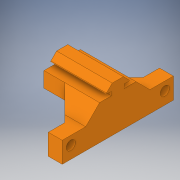
# Autodesk Inventor part: 20X20 lift conecter
Saved by Autodesk Inventor 2019 (Build 230136000, 136)
## iProperties
Created: 2018-10-23
Part Number: 20X20 lift conecter
Material: PC/ABS Plastic
Document SubType Name: Modeling
Designer: User
Density: 0.357273 g/cm^3
Appearance: Orange
Mass: 2.99758 g
Surface Area: 36.2331 cm^2
Volume: 8.39019 cm^3
Author: User
Autodesk Inventor part; units mm, degrees
ref_plane "YZ Plane" through (0, 0, 0) normal (1, 0, 0) x (0, 1, 0)
ref_plane "XZ Plane" through (0, 0, 0) normal (0, 1, 0) x (-1, 0, 0)
ref_plane "XY Plane" through (0, 0, 0) normal (0, 0, 1) x (1, 0, 0)
sketch "Sketch1" plane through (0, 0, 0) normal (0, 1, 0) x (-1, 0, 0)
  line L0 (2.54, 0) -> (5.715, 0)
  line L1 (5.715, 0) -> (5.715, -16.637)
  line L2 (5.715, -16.637) -> (2.54, -16.637)
  line L3 (2.54, -5.3975) -> (7.493, -5.3975)
  line L4 (7.493, -5.3975) -> (7.493, -11.2395)
  line L5 (7.493, -11.2395) -> (2.54, -11.2395)
  line L6 (10.5664, -5.7785) -> (10.5664, -10.8585)
  line L7 (7.493, -13.9319) -> (7.493, -2.7051)
  line L8 (7.493, -13.9319) -> (10.5664, -10.8585)
  line L9 (7.493, -2.7051) -> (10.5664, -5.7785)
  line L10 (2.54, -16.637) -> (2.54, 0)
  point P0 (0, 0)
  dimension "d1" = 16.637
  dimension "d2" = 1.778
  dimension "d9" = 3.0734
  dimension "d12" = 0
  dimension "d16" = 11.2268
  dimension "d20" = 135
  dimension "d21" = 135
  dimension "d26" = 2.6924
  dimension "d38" = 5.08
  dimension "d77" = 5.842
  dimension "d78" = 5.3975
  constraints: 22 end point, 3 parallel, 2 horizontal, 2 perpendicular, 2 point on line
  measures "d1" distance of L0.end L1.end
  measures "d2" distance between parallel lines of L4 L1
  measures "d9" distance between parallel lines of L6 L7
  measures "d12" distance between parallel lines of L4 L7
  measures "d16" distance of L7.start L7.end
  measures "d20" angle of L8 L6
  measures "d21" angle of L9 L6
  measures "d26" distance from line of L3 L7.end
  measures "d38" distance of L6.start L6.end
  measures "d77" distance between parallel lines of L5 L3
  measures "d78" distance between parallel lines of L2 L5
extrude "Extrusion2" add sketch "Sketch1" along normal blind 25.4
fillet "Fillet1" radius 0.254 2 edges at (-7.493, 12.7, -13.9319) (-7.493, 12.7, -2.7051)
thicken "Thicken1" operation add thickness 3.81 both sides no extend neighbours yes toward (1, 0, 0) faces at (-2.54, 8.4667, -5.5457)
sketch "Sketch2" plane through (0, 25.4, 0) normal (0, 1, 0) x (1, 0, 0)
  line L0 (-5.715, 5.3975) -> (-5.715, 0) projected
  line L1 (-5.715, 16.637) -> (-5.715, 11.2395) projected
  line L2 (-5.715, 0) -> (10.16, 0)
  line L3 (10.16, 0) -> (10.16, 16.637)
  line L4 (10.16, 16.637) -> (-5.715, 16.637)
  line L5 (-5.715, 16.637) -> (-5.715, 0)
  point P0 (0, 0)
  dimension "d46" = 15.875
  constraints: 8 end point, 2 parallel, 1 horizontal, 1 perpendicular
  measures "d46" distance of L4.end L3.end
extrude "Extrusion3" add sketch "Sketch2" against normal blind 6.35
sketch "Sketch3" plane through (0, 25.4, 0) normal (0, 1, 0) x (1, 0, 0)
  line L0 (0.635, -17.0815) -> (10.16, -17.0815)
  line L1 (10.16, -17.0815) -> (10.16, 33.7185)
  line L2 (10.16, 33.7185) -> (0.635, 33.7185)
  line L3 (0.635, 33.7185) -> (0.635, -17.0815)
  line L4 (10.16, 0) -> (10.16, 16.637) projected
  line L5 (-5.715, 11.2395) -> (-7.493, 11.2395) projected
  line L6 (-7.493, 11.2395) -> (-7.493, 13.3187) projected
  arc A0 (-7.493, 13.3187) -> (-7.9266, 13.4983) centre (-7.747, 13.3187) ccw projected
  line L7 (-7.9266, 13.4983) -> (-10.5664, 10.8585) projected
  line L8 (-10.5664, 10.8585) -> (-10.5664, 5.7785) projected
  line L9 (-10.5664, 5.7785) -> (-7.9266, 3.1387) projected
  arc A1 (-7.9266, 3.1387) -> (-7.493, 3.3183) centre (-7.747, 3.3183) ccw projected
  line L10 (-7.493, 3.3183) -> (-7.493, 5.3975) projected
  line L11 (-7.493, 5.3975) -> (-5.715, 5.3975) projected
  line L12 (-5.715, 5.3975) -> (-5.715, 0) projected
  line L13 (-5.715, 0) -> (10.16, 0) projected
  line L14 (10.16, 0) -> (10.16, 16.637) projected
  line L15 (10.16, 16.637) -> (-5.715, 16.637) projected
  line L16 (-5.715, 16.637) -> (-5.715, 11.2395) projected
  point P0 (0, 0)
  dimension "d49" = 50.8
  dimension "d50" = 16.637
  dimension "d51" = 17.0815
  dimension "d52" = 9.525
  constraints: 8 end point, 2 parallel, 1 collinear, 1 horizontal, 1 perpendicular
  measures "d49" distance of L0.end L1.end
  measures "d50" distance between parallel lines of L15 L13
  measures "d51" distance between parallel lines of L13 L0
  measures "d52" distance of L1.end L2.end
extrude "Extrusion4" add sketch "Sketch3" against normal blind 6.35 contours L3 L13 L1 L0 | L3 L15 L1 L13 | L3 L2 L1 L15
chamfer "Chamfer1" distance 6.35 angle 45 2 edges at (0.635, 22.225, 0) (0.635, 22.225, -16.637)
chamfer "Chamfer2" [suppressed]
chamfer "Chamfer3" distance 9.525 angle 45 4 edges at (0.9525, 19.05, 0) (-2.54, 19.05, 0) (-2.54, 19.05, -16.637) (0.9525, 19.05, -16.637)
sketch "Sketch4" plane through (0, 25.4, 0) normal (0, 1, 0) x (1, 0, 0)
  line L0 (0.635, -17.0815) -> (10.16, -17.0815) projected
  line L1 (10.16, -17.0815) -> (10.16, 33.7185) projected
  line L2 (10.16, 33.7185) -> (0.635, 33.7185) projected
  line L3 (0.635, 26.162) -> (0.635, 33.7185) projected
  line L4 (0.635, -17.0815) -> (0.635, -9.525) projected
  point P0 (0, 0)
  point P1 (4.5466, -13.1699)
  point P2 (4.5466, 29.8069)
  dimension "d64" = 3.9116
  dimension "d66" = 3.9116
  dimension "d75" = 3.9116
  dimension "d76" = 3.9116
  measures "d64" distance from line of L0 point (4.547, -13.17)
  measures "d66" distance from line of L2 point (4.547, 29.807)
  measures "d75" distance from line of L3 point (4.547, 29.807)
  measures "d76" distance from line of L4 point (4.547, -13.17)
hole "Hole1" at (4.5466, 25.4, 13.1699) at (4.5466, 25.4, -29.8069) direction (0, -1, 0) diameter 4.191 end through all
equation "\"d16\" = d15"
equation "\"d21\" = d20"
equation "\"d15\" = 11.2268"
body "Solid2"
